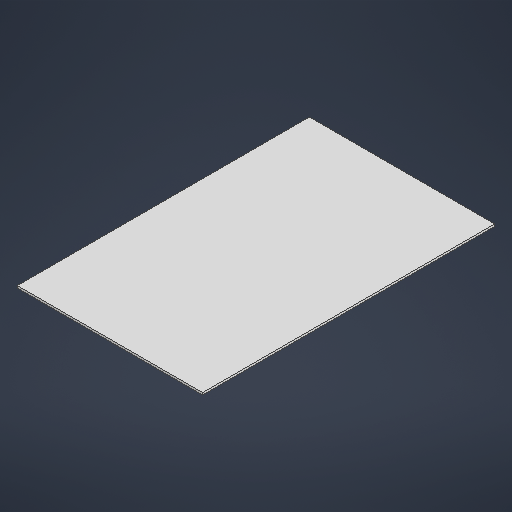
# Autodesk Inventor part: panel
Saved by Autodesk Inventor 2026.2 (Build 302298000, 298)
## iProperties
Created: 2026-01-05
Part Number: panel
Material: Genérico
Document SubType Name: Modeling
Designer: vicho
Density: 1 g/cm^3
Appearance: Valor por defecto
Author: vicho
Autodesk Inventor part; units mm, degrees
ref_plane "YZ Plane" through (0, 0, 0) normal (1, 0, 0) x (0, 1, 0)
ref_plane "XZ Plane" through (0, 0, 0) normal (0, 1, 0) x (-1, 0, 0)
ref_plane "XY Plane" through (0, 0, 0) normal (0, 0, 1) x (1, 0, 0)
sketch "Boceto1" plane through (0, 0, 0) normal (0, 0, 1) x (1, 0, 0)
  line L0 (173.5, -273.5) -> (-173.5, -273.5)
  line L1 (-173.5, -273.5) -> (-173.5, 273.5)
  line L2 (-173.5, 273.5) -> (173.5, 273.5)
  line L3 (173.5, 273.5) -> (173.5, -273.5)
  line L4 (173.5, -273.5) -> (-173.5, 273.5) construction
  line L5 (-173.5, -273.5) -> (173.5, 273.5) construction
  point P0 (0, 0)
  dimension "d0" = 347
  dimension "d1" = 547
  constraints: 12 end point, 2 midpoint, 2 parallel, 1 horizontal, 1 perpendicular
  measures "d0" distance between parallel lines of L3 L1
  measures "d1" distance between parallel lines of L0 L2
extrude "Extrusión1" add sketch "Boceto1" along normal blind 4
